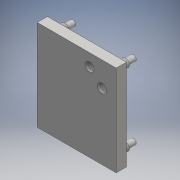
# Autodesk Inventor part: PCBMount
Saved by Autodesk Inventor 2016 (Build 200138000, 138)
## iProperties
Created: 2016-05-04
Part Number: PCBMount
Material: Generic
Document SubType Name: Modeling
Designer: mkepler
Density: 1 g/cm^3
Appearance: Default
Author: mkepler
Autodesk Inventor part; units mm, degrees
ref_plane "YZ Plane" through (0, 0, 0) normal (1, 0, 0) x (0, 1, 0)
ref_plane "XZ Plane" through (0, 0, 0) normal (0, 1, 0) x (-1, 0, 0)
ref_plane "XY Plane" through (0, 0, 0) normal (0, 0, 1) x (1, 0, 0)
sketch "Sketch1" plane through (0, 0, 0) normal (0, 1, 0) x (-1, 0, 0)
  line L0 (0, 0) -> (38.7, 0)
  line L1 (38.7, 0) -> (38.7, -44.5)
  line L2 (38.7, -44.5) -> (0, -44.5)
  line L3 (0, -44.5) -> (0, 0)
  line L4 (38.7, -22.25) -> (0, -22.25)
  line L5 (19.35, 0) -> (19.35, -44.5)
  dimension "d0" = 38.7
  dimension "d1" = 44.5
  constraints: 12 end point, 4 midpoint, 2 parallel, 1 horizontal, 1 perpendicular
  measures "d0" distance of L1.end L2.end
  measures "d1" distance of L0.end L1.end
extrude "Extrusion1" add sketch "Sketch1" along normal blind 5
sketch "Sketch2" plane through (0, 5, 0) normal (0, 1, 0) x (1, 0, 0)
  circle A0 centre (-34.2, 4.5) radius 2
  line L0 (-38.7, 0) -> (0, 0) projected
  line L1 (-38.7, 44.5) -> (-38.7, 0) projected
  circle A1 centre (-34.2, 40) radius 2
  line L2 (0, 44.5) -> (-38.7, 44.5) projected
  circle A2 centre (-4.5, 4.5) radius 2
  line L3 (0, 0) -> (0, 44.5) projected
  circle A3 centre (-4.5, 40) radius 2
  dimension "d16" = 4
  dimension "d17" = 4.5
  dimension "d18" = 4.5
  dimension "d19" = 4
  dimension "d20" = 4.5
  dimension "d21" = 4.5
  dimension "d22" = 4
  dimension "d23" = 4.5
  dimension "d24" = 4.5
  dimension "d25" = 4
  dimension "d26" = 4.5
  dimension "d27" = 4.5
  constraints: 4 centre point
  measures "d16" diameter of A0
  measures "d17" distance from line of L0 A0.centre
  measures "d18" distance from line of A0.centre L1
  measures "d19" diameter of A1
  measures "d20" distance from line of L1 A1.centre
  measures "d21" distance from line of A1.centre L2
  measures "d22" diameter of A2
  measures "d23" distance from line of L3 A2.centre
  measures "d24" distance from line of L0 A2.centre
  measures "d25" diameter of A3
  measures "d26" distance from line of A3.centre L2
  measures "d27" distance from line of L3 A3.centre
extrude "Extrusion2" add sketch "Sketch2" along normal blind 4 contours A0 | A1 | A2 | A3
sketch "Sketch3" plane through (-34.2, 9, -40) normal (0, 1, 0) x (1, 0, 0)
  circle A0 centre (0, 0) radius 1.35
  circle A1 centre (29.7, 0) radius 2 projected
  circle A2 centre (29.7, 0) radius 1.35
  circle A3 centre (29.7, -35.5) radius 2 projected
  circle A4 centre (29.7, -35.5) radius 1.35
  circle A5 centre (0, -35.5) radius 2 projected
  circle A6 centre (0, -35.5) radius 1.35
  point P0 (34.2, -40)
  dimension "d30" = 2.7
  dimension "d31" = 2.7
  dimension "d32" = 2.7
  dimension "d33" = 2.7
  constraints: 4 centre point, 3 coincident
  measures "d30" diameter of A0
  measures "d31" diameter of A2
  measures "d32" diameter of A4
  measures "d33" diameter of A6
extrude "Extrusion3" add sketch "Sketch3" along normal blind 4 contours A0 | A2 | A4 | A6
sketch "Sketch4" plane through (0, 0, 0) normal (0, -1, 0) x (1, 0, 0)
  circle A0 centre (-13, -6) radius 2.175
  line L0 (0, 0) -> (0, -44.5) projected
  line L1 (-38.7, 0) -> (0, 0) projected
  line L2 (-13, -6) -> (-13, -12)
  line L3 (-13, -12) -> (-7, -12)
  circle A1 centre (-7, -12) radius 2.175
  dimension "d36" = 4.35
  dimension "d37" = 13
  dimension "d38" = 6
  dimension "d39" = 6
  dimension "d40" = 6
  dimension "d41" = 4.35
  constraints: 4 end point, 2 centre point, 1 coincident, 1 perpendicular, 1 vertical
  measures "d36" diameter of A0
  measures "d37" distance from line of L0 L2.start
  measures "d38" distance from line of L2.start L1
  measures "d39" distance of L2.start L2.end
  measures "d40" distance of L2.end L3.end
  measures "d41" diameter of A1
hole "Hole1" at (-13, 0, -6) at (-7, 0, -12) direction (0, 1, 0) diameter 4.35 depth 4.5
body "Solid1"
